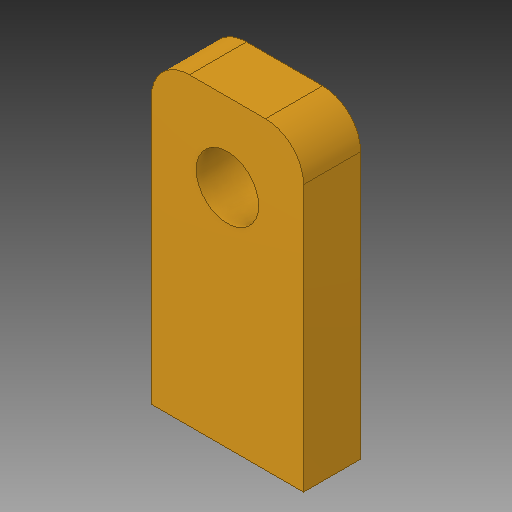
# Autodesk Inventor part: モーター端子
Saved by Autodesk Inventor 2018 (Build 220112000, 112)
## iProperties
Part Number: モーター端子
Material: 一般
Document SubType Name: Modeling
Designer: eieio
Density: 1 g/cm^3
Appearance: 溶接 - 真鍮
Author: eieio
Autodesk Inventor part; units mm, degrees
ref_plane "YZ Plane" through (0, 0, 0) normal (1, 0, 0) x (0, 1, 0)
ref_plane "XZ Plane" through (0, 0, 0) normal (0, 1, 0) x (-1, 0, 0)
ref_plane "XY Plane" through (0, 0, 0) normal (0, 0, 1) x (1, 0, 0)
sketch "スケッチ1" plane through (0, 0, 0) normal (0, 1, 0) x (-1, 0, 0)
  line L0 (0, 0) -> (4, 0)
  line L1 (4, 0) -> (4, -1.5)
  line L2 (4, -1.5) -> (0, -1.5)
  line L3 (0, -1.5) -> (0, 0)
  dimension "d0" = 4
  dimension "d1" = 1.5
  constraints: 8 end point, 2 parallel, 1 horizontal, 1 perpendicular
  measures "d0" distance between parallel lines of L3 L1
  measures "d1" distance between parallel lines of L2 L0
extrude "押し出し1" add sketch "スケッチ1" along normal blind 8
sketch "スケッチ2" plane through (-4, 0, 0) normal (0, 0, 1) x (1, 0, 0)
  circle A0 centre (2, 5.933) radius 0.8201
  line L0 (0, 0) -> (0, 8) projected
  point P0 (4, 0)
  dimension "d4" = 2
  constraints: 1 centre point
  measures "d4" distance from line of L0 A0.centre
extrude "押し出し2" cut sketch "スケッチ2" against normal blind 8
fillet "フィレット1" radius 1 2 edges at (0, 8, -0.75) (-4, 8, -0.75)
